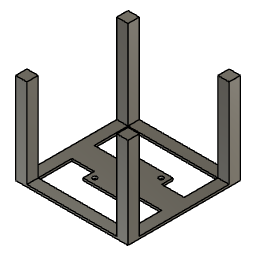
Imaging Sensor Bracket (Autodesk Fusion 360 design; units mm, degrees)
Autodesk Fusion 360 part; units mm, degrees
sketch "Sketch3" plane through (0, 0, 47) normal (0, 0, 1) x (-1, 0, 0)
  line L0 (-30, 30) -> (30, 30)
  line L1 (30, -30) -> (-30, -30)
  line L2 (-30, -30) -> (-30, 30)
  line L3 (40, 40) -> (-40, 40)
  line L4 (-40, 40) -> (-40, -40)
  line L5 (-40, -40) -> (40, -40)
  line L6 (40, -40) -> (40, 40)
  line L7 (-20, -20) -> (20, -20)
  line L8 (20, -20) -> (20, 20)
  line L9 (20, 20) -> (-20, 20)
  line L10 (-20, 20) -> (-20, -20)
  line L11 (-20, -20) -> (20, 20) construction
  line L12 (20, -20) -> (-20, 20) construction
  line L13 (50, -50) -> (-50, -50)
  line L14 (-50, -50) -> (-50, 50)
  line L15 (-50, 50) -> (50, 50)
  line L16 (50, 50) -> (50, -50)
  line L17 (50, -50) -> (-50, 50) construction
  line L18 (-50, -50) -> (50, 50) construction
  line L19 (50, 50) -> (40, 50)
  line L20 (40, 50) -> (40, 40)
  line L21 (40, 40) -> (50, 40)
  line L22 (50, 40) -> (50, 50)
  line L23 (50, -50) -> (40, -50)
  line L24 (40, -50) -> (40, -40)
  line L25 (40, -40) -> (50, -40)
  line L26 (50, -40) -> (50, -50)
  line L27 (-50, -50) -> (-40, -50)
  line L28 (-40, -50) -> (-40, -40)
  line L29 (-40, -40) -> (-50, -40)
  line L30 (-50, -40) -> (-50, -50)
  line L31 (-40, 40) -> (-50, 40)
  line L32 (-50, 40) -> (-50, 50)
  line L33 (-50, 50) -> (-40, 50)
  line L34 (-40, 50) -> (-40, 40)
  circle A0 centre (0, 0) radius 35
  line L35 (-50, -10) -> (50, -10)
  line L36 (50, -10) -> (50, 10)
  line L37 (50, 10) -> (-50, 10)
  line L38 (-50, 10) -> (-50, -10)
  line L39 (-50, -10) -> (50, 10) construction
  line L40 (50, -10) -> (-50, 10) construction
  dimension "d15" = 40
  dimension "d16" = 40
  dimension "d18" = 100
  dimension "d19" = 100
  dimension "d28" = 70
  dimension "d29" = 20
  constraint perpendicular L7 L8
  constraint parallel L7 L9
  constraint parallel L8 L10
  constraint horizontal L7
  constraint coincident L11 A0.centre
  constraint coincident L12 A0.centre
  constraint coincident A0.centre origin
  constraint perpendicular L13 L14
  constraint parallel L13 L15
  constraint parallel L14 L16
  constraint horizontal L13
  constraint coincident L17 A0.centre
  constraint coincident L18 A0.centre
  constraint horizontal L19
  constraint vertical L20
  constraint horizontal L21
  constraint vertical L22
  constraint coincident L3.start L6.end
  constraint horizontal L23
  constraint vertical L24
  constraint horizontal L25
  constraint vertical L26
  constraint coincident L5.end L6.start
  constraint horizontal L27
  constraint vertical L28
  constraint horizontal L29
  constraint vertical L30
  constraint coincident L4.end L5.start
  constraint horizontal L31
  constraint vertical L32
  constraint horizontal L33
  constraint vertical L34
  constraint coincident L3.end L4.start
  constraint perpendicular L35 L36
  constraint parallel L35 L37
  constraint parallel L36 L38
  constraint horizontal L35
  constraint coincident L39 A0.centre
  constraint coincident L40 A0.centre
  measures "d15" distance of L8.end L9.end
  measures "d16" distance of L7.end L8.end
  measures "d18" distance of L14.end L15.end
  measures "d19" distance of L13.end L14.end
  measures "d28" diameter of A0
  measures "d29" distance of L35.end L36.end
extrude "Extrude3" add sketch "Sketch3" against normal blind 50 contours L14 L15 L31 L32 L33 L34 | L15 L16 L19 L20 L21 L22 | L13 L14 L27 L28 L29 L30 | L13 L16 L23 L24 L25 L26 makes body 1 at (-43.3333, 40, 30.3333) makes body 2 at (43.3333, 50, 30.3333) makes body 3 at (-43.3333, -50, 30.3333) makes body 4 at (43.3333, -40, 30.3333)
extrude "Extrude4" cut 4 faces at (46.6667, 43.3333, 47) (-43.3333, 43.3333, 47) (43.3333, -43.3333, 47) (-43.3333, -46.6667, 47) along direction (0, 0, -1) blind 2 on bodies 1 2 3 4 bodies 1 2 3 4
extrude "Extrude5" cut 4 faces at (-43.3333, 43.3333, -3) (46.6667, 43.3333, -3) (43.3333, -43.3333, -3) (-43.3333, -46.6667, -3) along direction (0, 0, 1) blind 3 on bodies 1 2 3 4 bodies 1 2 3 4
extrude "Extrude6" add sketch "Sketch3" against normal blind 2 contours L4 L14 L31 L37 | L4 L14 L35 L37 L38 | L6 L16 L35 L36 L37 | L6 L16 L21 L37 | L4 L14 L29 L35 | L3 L15 L20 L34 | L14 L15 L31 L32 L33 L34 | L6 L16 L25 L35 | L15 L16 L19 L20 L21 L22 | L5 L13 L24 L28 | L13 L14 L27 L28 L29 L30 | L13 L16 L23 L24 L25 L26 bodies 1 2 3 4
sketch "Sketch4" plane through (0, 0, 0) normal (0, 0, 1) x (1, 0, 0)
extrude "Extrude7" add sketch "Sketch3" against normal blind 2 contours L2 L10 L35 L37 | L2 A0 L35 L37 | L4 A0 L35 L37 | L6 A0 L35 L37 | L8 A0 L35 L37 | L8 L10 L35 L37 | L8 L9 L10 L37 | L7 L8 L10 L35 bodies 1
sketch "Sketch5" plane through (0, 0, 47) normal (0, 0, 1) x (-1, 0, 0)
  line L0 (-20, 20) -> (-16, 20)
  line L1 (-16, 20) -> (-16, 16)
  circle A0 centre (-16, 16) radius 2
  line L2 (20, 20) -> (-20, 20)
  line L3 (0, 20) -> (0, -20)
  line L4 (50, 40) -> (50, -40)
  line L5 (-50, -40) -> (-50, 40)
  line L6 (50, 0) -> (-50, 0)
  circle A1 centre (16, 16) radius 2
  circle A2 centre (-16, -16) radius 2
  circle A3 centre (16, -16) radius 2
  point P0 (-20, 20)
  dimension "d32" = 4
  dimension "d33" = 4
  constraint coincident P0 L0.start
  constraint perpendicular L0 L1
  constraint coincident L1.end A0.centre
  constraint midpoint L2 L3.start
  constraint perpendicular L2 L3
  constraint midpoint L4 L6.start
  constraint midpoint L5 L6.end
  constraint symmetric A0 L3 A1
  constraint symmetric A0 L6 A2
  constraint symmetric L6 A1 A3
  measures "d32" distance of P0 L0.end
  measures "d33" diameter of A0
extrude "Extrude8" cut sketch "Sketch5" against normal blind 6 bodies 1
sketch "Sketch6" plane through (0, 0, 47) normal (0, 0, 1) x (-1, 0, 0)
  circle A0 centre (16, 16) radius 2
  circle A1 centre (16, -16) radius 2
  circle A2 centre (-16, 16) radius 2
  circle A3 centre (-16, -16) radius 2
  line L0 (-40, 10) -> (-40, 40)
  line L1 (-40, 40) -> (40, 40)
  line L2 (40, 40) -> (40, 10)
  line L3 (40, 10) -> (20, 10)
  line L4 (20, 10) -> (20, 20)
  line L5 (20, 20) -> (-20, 20)
  line L6 (-20, 20) -> (-20, 10)
  line L7 (-20, 10) -> (-40, 10)
  line L8 (-40, -10) -> (-20, -10)
  line L9 (-20, -10) -> (-20, -20)
  line L10 (-20, -20) -> (20, -20)
  line L11 (20, -20) -> (20, -10)
  line L12 (20, -10) -> (40, -10)
  line L13 (40, -10) -> (40, -40)
  line L14 (40, -40) -> (-40, -40)
  line L15 (-40, -40) -> (-40, -10)
  line L16 (-50, 50) -> (-50, -50)
  line L17 (-50, -50) -> (50, -50)
  line L18 (50, -50) -> (50, 50)
  line L19 (50, 50) -> (-50, 50)
  line L20 (16, -16) -> (14.75, -16)
  line L21 (14.75, -16) -> (14.75, -14.75)
  line L22 (0, -20) -> (0, 20)
  line L23 (20, 0) -> (-20, 0)
  circle A4 centre (14.75, -14.75) radius 2
  circle A5 centre (-14.75, -14.75) radius 2
  circle A6 centre (14.75, 14.75) radius 2
  circle A7 centre (-14.75, 14.75) radius 2
  dimension "d36" = 1.25
  dimension "d37" = 1.25
  dimension "d38" = 4
  constraint coincident A1.centre L20.start
  constraint horizontal L20
  constraint perpendicular L20 L21
  constraint midpoint L10 L22.start
  constraint midpoint L5 L22.end
  constraint perpendicular L22 L23
  constraint coincident L21.end A4.centre
  constraint symmetric L22 A4 A5
  constraint symmetric L23 A4 A6
  constraint symmetric L23 A5 A7
  measures "d36" distance of A1.centre L20.end
  measures "d37" distance of L20.end L21.end
  measures "d38" diameter of A4
extrude "Extrude9" add sketch "Sketch6" against normal blind 2 contours A0 A6 | A0 A6 | A1 A4 | A1 A4 | A2 A7 | A2 A7 | A3 A5 | A3 A5 picked at (17.235, 16.6868) picked at (15.1398, 15.0878) picked at (17.235, -16.6868) picked at (15.1398, -15.0878) picked at (-15.6102, 15.6622) picked at (-16.5783, 16.5783) picked at (-15.6102, -15.6622) picked at (-16.5783, -16.5783) bodies 1
extrude "Extrude10" cut sketch "Sketch6" against normal blind 2 contours A0 A6 | A0 A6 | A1 A4 | A1 A4 | A2 A7 | A2 A7 | A3 A5 | A3 A5 picked at (15.1398, 15.0878) picked at (14.1717, 14.1717) picked at (15.1398, -15.0878) picked at (14.1717, -14.1717) picked at (-15.6102, 15.6622) picked at (-13.515, 14.0632) picked at (-15.6102, -15.6622) picked at (-13.515, -14.0632) bodies 1
move_body "Move1" bodies 1 to x (-1, 0, 0) y (0, 1, 0) z (0, 0, -1) at (100, 0, 94)
extrude "Extrude11" add 4 faces at (143.3333, 46.6667, 94) (143.3333, -46.6667, 94) (56.6667, -43.3333, 94) (53.3333, 43.3333, 94) along direction (0, 0, 1) blind 34 on bodies 1 bodies 1
move_body "Move2" bodies 1 to x (1, 0, 0) y (0, 1, 0) z (0, 0, 1) at (-100, 0, -47)
